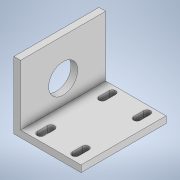
# Autodesk Inventor part: Big Motor Bracket
Saved by Autodesk Inventor 2022 (Build 260153000, 153)
## iProperties
Created: 2021-06-03
Part Number: Big Motor Bracket
Material: Generic
Document SubType Name: Modeling
Designer: jrcol
Density: 1 g/cm^3
Appearance: Default
Author: jrcol
Autodesk Inventor part; units mm, degrees
ref_plane "YZ Plane" through (0, 0, 0) normal (1, 0, 0) x (0, 1, 0)
ref_plane "XZ Plane" through (0, 0, 0) normal (0, 1, 0) x (-1, 0, 0)
ref_plane "XY Plane" through (0, 0, 0) normal (0, 0, 1) x (1, 0, 0)
sketch "Sketch1" plane through (0, 0, 0) normal (0, 1, 0) x (-1, 0, 0)
  line L0 (0, 0) -> (30, 0)
  line L1 (30, 0) -> (30, 38)
  line L2 (30, 38) -> (0, 38)
  line L3 (0, 38) -> (0, 0)
  dimension "d0" = 38
  dimension "d1" = 30
  constraints: 8 end point, 2 parallel, 1 horizontal, 1 perpendicular
  measures "d0" distance of L0.end L1.end
  measures "d1" distance of L1.end L2.end
extrude "Extrusion1" add sketch "Sketch1" along normal blind 3
sketch "Sketch2" plane through (0, 3, 0) normal (0, 1, 0) x (1, 0, 0)
  line L0 (-30, 0) -> (-30, -38) projected
  line L1 (0, 0) -> (-30, 0) projected
  line L2 (-30, -38) -> (-27, -38)
  line L3 (-27, -38) -> (-27, 0)
  line L4 (-27, 0) -> (-30, 0)
  line L5 (-30, 0) -> (-30, -38)
  dimension "d4" = 3
  constraints: 8 end point, 2 parallel, 1 horizontal, 1 perpendicular, 1 point on line
  measures "d4" distance of L0.end L2.end
extrude "Extrusion2" add sketch "Sketch2" along normal blind 27
sketch "Sketch3" plane through (-27, 3, 38) normal (1, 0, 0) x (0, 0, -1)
  circle A0 centre (19, 10.5) radius 6.5
  line L0 (38, 27) -> (0, 27) projected
  point P0 (38, -3)
  dimension "d7" = 13
  dimension "d8" = 16.5
  constraints: 1 centre point
  measures "d7" diameter of A0
  measures "d8" distance from line of L0 A0.centre
extrude "Extrusion3" cut sketch "Sketch3" against normal up to surface (3 mm away)
sketch "Sketch4" plane through (0, 3, 0) normal (0, 1, 0) x (1, 0, 0)
  line L0 (0, 0) -> (-30, 0) projected
  line L1 (-27, -38) -> (-27, 0) projected
  line L2 (-27, -19) -> (0, -19) construction
  line L3 (-5.5, -35) -> (-5.5, -30.5) construction
  line L4 (-4, -35) -> (-4, -30.5)
  line L5 (-7, -30.5) -> (-7, -35)
  arc A0 (-7, -35) -> (-4, -35) centre (-5.5, -35) ccw
  arc A1 (-4, -30.5) -> (-7, -30.5) centre (-5.5, -30.5) ccw
  line L6 (-27, -38) -> (0, -38) projected
  line L7 (-5.5, -7.5) -> (-5.5, -3) construction
  line L8 (-7, -7.5) -> (-7, -3)
  line L9 (-4, -3) -> (-4, -7.5)
  arc A2 (-7, -7.5) -> (-4, -7.5) centre (-5.5, -7.5) ccw
  arc A3 (-4, -3) -> (-7, -3) centre (-5.5, -3) ccw
  line L10 (0, -38) -> (0, 0) projected
  line L11 (-4, -3) -> (-21, -3) construction
  line L12 (-21, -3) -> (-21, -7.5) construction
  line L13 (-22.5, -3) -> (-22.5, -7.5)
  line L14 (-19.5, -7.5) -> (-19.5, -3)
  arc A4 (-19.5, -3) -> (-22.5, -3) centre (-21, -3) ccw
  arc A5 (-22.5, -7.5) -> (-19.5, -7.5) centre (-21, -7.5) ccw
  line L15 (-21.1462, -34.8538) -> (-21.1462, -30.3538) construction
  line L16 (-22.7923, -34.8538) -> (-22.7923, -30.3538)
  line L17 (-19.5, -30.3538) -> (-19.5, -34.8538)
  arc A6 (-22.7923, -34.8538) -> (-19.5, -34.8538) centre (-21.1462, -34.8538) ccw
  arc A7 (-19.5, -30.3538) -> (-22.7923, -30.3538) centre (-21.1462, -30.3538) ccw
  point P0 (-5.5, -32.75)
  point P1 (-5.5, -5.25)
  point P2 (-21, -5.25)
  point P3 (-21.1462, -32.6038)
  dimension "d11" = 1.5
  dimension "d12" = 7.5
  dimension "d13" = 3
  dimension "d14" = 1.5
  dimension "d15" = 3
  dimension "d16" = 7.5
  dimension "d17" = 4
  dimension "d18" = 17
  dimension "d19" = 3
  dimension "d20" = 7.5
  dimension "d21" = 1.5
  constraints: 36 end point, 16 point on circle, 16 tangent, 8 centre point, 5 midpoint, 4 parallel, 4 vertical, 2 collinear, 2 horizontal
  measures "d11" distance edge to line of A0 L6
  measures "d13" distance between parallel lines of L5 L4
  measures "d14" distance edge to line of A3 L0
  measures "d15" distance between parallel lines of L8 L9
  measures "d17" distance between parallel lines of L10 L4
  measures "d18" distance of L9.start L11.end
  measures "d19" distance between parallel lines of L14 L13
  measures "d21" distance edge to line of A6 L6
extrude "Extrusion4" cut sketch "Sketch4" against normal through all contours A0 L5 A1 L4 | L8 A3 L9 A2 | A4 L14 A5 L13 | L16 A7 L17 A6
equation "\"d14\" = d11"
equation "\"d15\" = d13"
equation "\"d16\" = d12"
equation "\"d19\" = d13"
body "Solid1"
